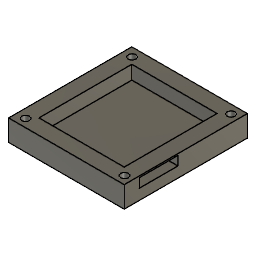
SmartClockBottom (Autodesk Fusion 360 design; units mm, degrees)
part number: 2026-04-05-15-54-36-238
Autodesk Fusion 360 part; units mm, degrees
sketch "Sketch1" plane through (0, 0, 0) normal (0, 0, 1) x (1, 0, 0)
  line L0 (-0.9, 0.7) -> (53.1, 0.7)
  line L1 (53.1, 0.7) -> (53.1, -60.3)
  line L2 (53.1, -60.3) -> (-0.9, -60.3)
  line L3 (-0.9, -60.3) -> (-0.9, 0.7)
  line L4 (-10.9, 10.7) -> (63.1, 10.7)
  line L5 (63.1, 10.7) -> (63.1, -70.3)
  line L6 (63.1, -70.3) -> (-10.9, -70.3)
  line L7 (-10.9, -70.3) -> (-10.9, 10.7)
  dimension "d2" = 61
  dimension "d3" = 54
  dimension "d4" = 81
  dimension "d5" = 74
  dimension "d6" = 10
  dimension "d7" = 10
  constraint horizontal L0
  constraint vertical L1
  constraint horizontal L2
  constraint vertical L3
  constraint horizontal L4
  constraint vertical L5
  constraint horizontal L6
  constraint vertical L7
  measures "d2" distance of L0.start L2.end
  measures "d3" distance of L0.start L0.end
  measures "d4" distance of L4.start L6.end
  measures "d5" distance of L4.start L4.end
  measures "d6" distance of L1 L5
  measures "d7" distance of L2 L6
extrude "Extrude1" add sketch "Sketch1" along normal blind 5 contours L0 L1 L2 L3
extrude "Extrude2" add sketch "Sketch1" along normal blind 15
sketch "Sketch2" plane through (53.1, 0, 0) normal (-1, 0, 0) x (0, -1, 0)
  line L0 (-0.7, 5) -> (60.3, 5)
  line L1 (60.3, 5) -> (60.3, 15)
  line L2 (60.3, 15) -> (-0.7, 15)
  line L3 (-0.7, 15) -> (-0.7, 5)
  line L4 (48, 11) -> (60.3, 11)
  line L5 (60.3, 11) -> (60.3, 5)
  line L6 (60.3, 5) -> (48, 5)
  line L7 (48, 5) -> (48, 11)
  constraint horizontal L4
  constraint vertical L5
  constraint horizontal L6
  constraint vertical L7
  constraint coincident L0.end L1.start
extrude "Extrude3" cut sketch "Sketch2" against normal blind 18 contours L0 L1 L4 L5 L6 L7
sketch "Sketch3" plane through (0, 0, 15) normal (0, 0, 1) x (-1, 0, 0)
  line L0 (-53.1, 60.3) -> (0.9, 60.3)
  line L1 (0.9, 60.3) -> (0.9, -0.7)
  line L2 (0.9, -0.7) -> (-53.1, -0.7)
  line L3 (-53.1, -0.7) -> (-53.1, 60.3)
  line L4 (10.9, 70.3) -> (-63.1, 70.3)
  line L5 (-63.1, 70.3) -> (-63.1, -10.7)
  line L6 (-63.1, -10.7) -> (10.9, -10.7)
  line L7 (10.9, -10.7) -> (10.9, 70.3)
  circle A0 centre (5, -5) radius 2.5
  circle A1 centre (-58, -5) radius 2.5
  circle A2 centre (5, 65) radius 2.5
  circle A3 centre (-58, 65) radius 2.5
  dimension "d14" = 5
  dimension "d15" = 5
  dimension "d16" = 5
  dimension "d17" = 5
  measures "d14" diameter of A0
  measures "d15" diameter of A1
  measures "d16" diameter of A2
  measures "d17" diameter of A3
extrude "Extrude4" cut sketch "Sketch3" against normal blind 20 contours A0 | A1 | A2 | A3
extrude "Extrude5" cut 1 faces at (56.4333, -48, 7) along direction (0, 1, 0) blind 10
move_face "MoveFace1" to x (1, 0, 0) y (0, 1, 0) z (0, 0, 1) at (-2, 0, 0) 2 faces at (-7.4876, -64.7511, 5) (-7.4876, 5.2489, 5)
extrude "Extrude6" cut 1 faces at (-0.9, -39.9667, 8.3333) along direction (-1, 0, 0) blind 2
extrude "Extrude7" add 1 faces at (-10.9, -43.3, 5) along direction (-1, 0, 0) blind 2
sketch "Sketch4" plane through (0, 0, 5) normal (0, 0, 1) x (-1, 0, 0)
  line L0 (2.9, 60.3) -> (-63.1, 60.3)
  line L1 (-63.1, 60.3) -> (-63.1, 38)
  line L2 (-63.1, 38) -> (-53.1, 38)
  line L3 (-53.1, 38) -> (-53.1, -0.7)
  line L4 (-53.1, -0.7) -> (2.9, -0.7)
  line L5 (2.9, -0.7) -> (2.9, 60.3)
  line L6 (-63.1, 38) -> (-52.9998, 38)
  line L7 (-52.9998, 38) -> (-52.9998, 60.3)
  line L8 (-52.9998, 60.3) -> (-63.1, 60.3)
  line L9 (-63.1, 60.3) -> (-63.1, 38)
  constraint horizontal L6
  constraint vertical L7
  constraint horizontal L8
  constraint vertical L9
  constraint coincident L0 L7.end
  constraint coincident L1.end L2.start
extrude "Extrude8" add sketch "Sketch4" along normal blind 2 contours L0 L1 L2 L6 L7 L8 L9
extrude "Extrude9" cut 1 faces at (56.4333, -38, 8.3333) along direction (0, 1, 0) blind 3
extrude "Extrude10" cut 1 faces at (56.4333, -51.8667, 11) along direction (0, 0, 1) blind 2
sketch "Sketch5" plane through (0, 0, 0) normal (0, 0, 1) x (1, 0, 0)
  line L0 (75, 10) -> (149, 10)
  line L1 (149, 10) -> (149, -71)
  line L2 (149, -71) -> (75, -71)
  line L3 (75, -71) -> (75, 10)
  dimension "d32" = 81
  dimension "d33" = 74
  constraint horizontal L0
  constraint vertical L1
  constraint horizontal L2
  constraint vertical L3
  measures "d32" distance of L0.start L2.end
  measures "d33" distance of L0.start L0.end
sketch "Sketch6" plane through (0, 0, 3) normal (0, 0, 1) x (-1, 0, 0)
  line L0 (-75, 71) -> (-149, 71)
  line L1 (-149, 71) -> (-149, -10)
  line L2 (-149, -10) -> (-75, -10)
  line L3 (-75, -10) -> (-75, 71)
  line L4 (-85, 0) -> (-139, 0)
  line L5 (-139, 0) -> (-139, 61)
  line L6 (-139, 61) -> (-85, 61)
  line L7 (-85, 61) -> (-85, 0)
  line L8 (-90, 5) -> (-115, 5)
  line L9 (-115, 5) -> (-115, 21.3718)
  line L10 (-115, 21.3718) -> (-90, 21.3718)
  line L11 (-90, 21.3718) -> (-90, 5)
  line L12 (-120, 5) -> (-135, 5)
  line L13 (-135, 5) -> (-135, 20)
  line L14 (-135, 20) -> (-120, 20)
  line L15 (-120, 20) -> (-120, 5)
  dimension "d36" = 61
  dimension "d37" = 54
  dimension "d38" = 10
  constraint horizontal L4
  constraint vertical L5
  constraint horizontal L6
  constraint vertical L7
  constraint horizontal L8
  constraint vertical L9
  constraint horizontal L10
  constraint vertical L11
  constraint horizontal L12
  constraint vertical L13
  constraint horizontal L14
  constraint vertical L15
  measures "d36" distance of L4.start L6.end
  measures "d37" distance of L4.start L4.end
  measures "d38" distance of L1 L5
extrude "Extrude21" cut 1 faces at (56.9756, -40.1, 15) along direction (0, 0, -1) blind 1
sketch "Sketch7" plane through (0, 0, 14) normal (0, 0, 1) x (-1, 0, 0)
  line L0 (12.9, 70.3) -> (-63.1, 70.3)
  line L1 (-63.1, 70.3) -> (-63.1, -10.7)
  line L2 (-63.1, -10.7) -> (12.9, -10.7)
  line L3 (12.9, -10.7) -> (12.9, 70.3)
  line L4 (-53.1, 60.3) -> (2.9, 60.3)
  line L5 (2.9, 60.3) -> (2.9, -0.7)
  line L6 (2.9, -0.7) -> (-53.1, -0.7)
  line L7 (-53.1, -0.7) -> (-53.1, 60.3)
  circle A0 centre (-58, -5) radius 2.5
  circle A1 centre (-58, 65) radius 2.5
  circle A2 centre (7, -5) radius 2.5
  circle A3 centre (7, 65) radius 2.5
  circle A4 centre (-142.9365, -5) radius 2.5
  circle A5 centre (-77.9365, -5) radius 2.5
  circle A6 centre (-77.9365, 65) radius 2.5
  circle A7 centre (-142.9365, 65) radius 2.5
